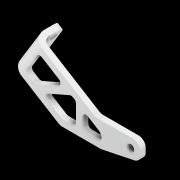
# Autodesk Inventor part: UpperArmActuatorBracket
Saved by Autodesk Inventor 2020 (Build 240168000, 168)
## iProperties
Created: 2020-04-16
Part Number: UpperArmActuatorBracket
Material: Aluminum 6061
Document SubType Name: Sheet Metal
Designer: valer
Density: 2.7 g/cm^3
Sheet Metal Rule: Default
Appearance: Aluminum - Flat
Author: valer
Autodesk Inventor part; units mm, degrees
ref_plane "YZ Plane" through (0, 0, 0) normal (1, 0, 0) x (0, 1, 0)
ref_plane "XZ Plane" through (0, 0, 0) normal (0, 1, 0) x (-1, 0, 0)
ref_plane "XY Plane" through (0, 0, 0) normal (0, 0, 1) x (1, 0, 0)
sketch "Base" plane through (0, 0, 0) normal (0, 0, 1) x (1, 0, 0)
  circle A0 centre (10.7322, 5.946) radius 3.175
  line L0 (19.1988, -0.9432) -> (19.1988, 14.4127)
  line L1 (19.1988, 14.4127) -> (-21.4412, 14.4127)
  line L2 (-21.4412, 14.4127) -> (-75.2998, 47.4242)
  line L3 (-75.2998, 47.4242) -> (-94.2145, 16.5647) construction
  line L4 (-94.2145, 16.5647) -> (-53.6099, -8.3231)
  line L5 (-73.288, 39.0412) -> (-85.8315, 18.5765)
  line L6 (-85.8315, 18.5765) -> (-76.5069, 12.8611)
  line L7 (-70.162, 8.9722) -> (-51.8903, -2.2271)
  line L8 (-73.288, 39.0412) -> (-49.6339, 24.5428)
  line L9 (-76.5069, 12.8611) -> (-49.6339, 24.5428)
  line L10 (-70.162, 8.9722) -> (-43.289, 20.6539)
  line L11 (-43.289, 20.6539) -> (-39.1903, 18.1417)
  line L12 (-33.0943, 14.4053) -> (-17.5079, 4.8519)
  line L13 (-17.5079, 4.8519) -> (-13.584, -2.2271)
  line L14 (-33.0943, 14.4053) -> (-33.0943, -2.2271)
  line L15 (-39.1903, 18.1417) -> (-39.1903, -2.2271)
  line L16 (-51.8903, -2.2271) -> (-39.1903, -2.2271)
  line L17 (-33.0943, -2.2271) -> (-13.584, -2.2271)
  line L18 (-53.6099, -8.3231) -> (-16.3415, -8.3231)
  line L19 (-94.2145, 16.5647) -> (-97.4629, 18.5557)
  line L20 (-97.4629, 18.5557) -> (-78.5481, 49.4153)
  line L21 (-78.5481, 49.4153) -> (-75.2998, 47.4242)
  line L22 (-16.3415, -8.3231) -> (19.1988, -0.9432)
  point P0 (0, 0)
  dimension "d0" = 6.35
  dimension "d1" = 6.096
  dimension "d2" = 6.096
  dimension "d3" = 6.096
  dimension "d4" = 6.096
  dimension "d5" = 6.096
  dimension "d6" = 6.096
  dimension "d7" = 55
  dimension "d8" = 61
  dimension "d11" = 47.625
  dimension "d12" = 36.195
  dimension "d17" = 10.9368
  dimension "d18" = 6.096
  dimension "d19" = 12.7
  dimension "d21" = 14.2691
  dimension "d22" = 8.4667
  dimension "d23" = 3.81
  dimension "d52" = 8.4667
  dimension "d54" = 8.4667
  dimension "d55" = 40.64
  measures "d0" diameter of A0
  measures "d1" distance between parallel lines of L14 L15
  measures "d2" distance between parallel lines of L2 L12
  measures "d3" distance between parallel lines of L18 L17
  measures "d4" distance between parallel lines of L2 L11
  measures "d5" distance between parallel lines of L4 L7
  measures "d6" distance between parallel lines of L3 L5
  measures "d7" angle of L10 L4
  measures "d8" angle of L18 L13
  measures "d11" distance of L3.end L4.end
  measures "d12" distance of L2.end L3.end
  measures "d17" distance of L5.end L6.end
  measures "d18" distance between parallel lines of L9 L10
  measures "d19" distance of L7.end L15.end
  measures "d21" distance from line of L18 A0.centre
  measures "d22" distance from line of L1 A0.centre
  measures "d23" distance of L3.end L19.end
  measures "d52" distance from line of L22 A0.centre
  measures "d54" distance from line of L0 A0.centre
  measures "d55" distance of L0.end L1.end
extrude "Plate1" add sketch "Base" along normal blind 5.08
sketch "Sketch3" plane through (-74.217, 46.7606, 5.08) normal (-0.8525909, 0.522579, 0) x (-0.522579, -0.8525909, 0)
  line L0 (36.195, 0) -> (0, 0)
  line L1 (0, 0) -> (0, -25.4)
  line L2 (0, -25.4) -> (36.195, -25.4)
  line L3 (36.195, -25.4) -> (36.195, 0)
  constraints: 6 end point, 1 horizontal, 1 perpendicular, 1 vertical
edge flange "Flange1" height 25.4 angle 90 thickness 5.08 bend radius 5.08 thickness toward (-0.8525909, 0.522579, 0) relief straight relief width 5.08 relief depth 2.54 edges at (-88.0055, 33.9855, 0) wall of the first edge with corners at (-93.1317, 15.901, 5.08) (-74.217, 46.7606, 5.08) (-74.217, 46.7606, -20.32) (-93.1317, 15.901, -20.32)
bend "Bend1"
corner "Corner1"
sketch "Sketch4" plane through (-93.1317, 15.901, -5.08) normal (0.8525909, -0.522579, 0) x (0, 0, -1)
  line L0 (0, 36.195) -> (0, 0) construction
  line L1 (0, 0) -> (15.24, 0) construction
  line L2 (15.24, 0) -> (15.24, 36.195) construction
  line L3 (0, 36.195) -> (15.24, 36.195) construction
  line L4 (15.24, 36.195) -> (0, 36.195) construction
  line L5 (8.89, 36.195) -> (8.89, 0) construction
  line L6 (0, 0) -> (15.24, 0) construction
  circle A0 centre (8.89, 27.7283) radius 3.175
  circle A1 centre (8.89, 8.6783) radius 3.175
  point P0 (-5.08, 35.1116)
  dimension "d38" = 6.35
  dimension "d39" = 6.35
  dimension "d40" = 6.35
  dimension "d41" = 8.4667
  dimension "d42" = 19.05
  constraints: 4 point on line, 2 centre point, 2 end point, 1 perpendicular
  measures "d38" diameter of A0
  measures "d39" diameter of A1
  measures "d40" distance between parallel lines of L2 L5
  measures "d41" distance from line of L3 A0.centre
  measures "d42" distance of A0.centre A1.centre
hole "Hole1" at (-78.6415, 39.542, -13.97) at (-88.5966, 23.3001, -13.97) direction (-0.8525909, 0.522579, 0) diameter 6.35 end through all
fillet "Fillet1" radius 6.35 7 edges at (19.1988, -0.9432, 2.54) (19.1988, 14.4127, 2.54) (-21.4412, 14.4127, 2.54) (-53.6099, -8.3231, 2.54) (-95.2973, 17.2284, -20.32) (-76.3826, 48.0879, -20.32) (-16.3415, -8.3231, 2.54)
fillet "Fillet2" radius 3.175 13 edges at (-49.6339, 24.5428, 2.54) (-76.5069, 12.8611, 2.54) (-43.289, 20.6539, 2.54) (-39.1903, 18.1417, 2.54) (-39.1903, -2.2271, 2.54) (-51.8903, -2.2271, 2.54) (-70.162, 8.9722, 2.54) (-33.0943, -2.2271, 2.54) (-13.584, -2.2271, 2.54) (-33.0943, 14.4053, 2.54) (-17.5079, 4.8519, 2.54) (-85.6149, 18.4437, 2.54) (-73.0715, 38.9085, 2.54)
equation "\"d48\" = Thickness"
equation "\"d25\" = Thickness"
equation "\"d28\" = BendReliefWidth"
equation "\"d29\" = BendReliefDepth"
equation "\"d30\" = MinimumRemnant"
equation "\"d31\" = TransitionRadius"
equation "\"d34\" = BendRadius"
equation "\"d35\" = CornerReliefSize"
equation "\"d36\" = GapSize"
equation "\"d37\" = JacobiRadiusSize"
equation "\"BendRadius\" = Thickness"
equation "\"BendReliefWidth\" = Thickness"
equation "\"BendReliefDepth\" = 0.5 * Thickness"
equation "\"CornerReliefSize\" = 4 * Thickness"
equation "\"MinimumRemnant\" = 2 * Thickness"
equation "\"TransitionRadius\" = BendRadius"
equation "\"JacobiRadiusSize\" = BendRadius"
equation "\"GapSize\" = Thickness"
equation "\"Thickness\" = 5.08"
body "Solid1"
